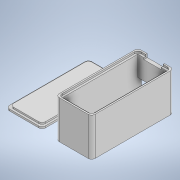
# Autodesk Inventor part: case
Saved by Autodesk Inventor 2021 (Build 250183000, 183)
## iProperties
Created: 2021-06-14
Part Number: case
Material: 일반
Document SubType Name: Modeling
Designer: dltjd
Density: 1 g/cm^3
Appearance: 기본값
Author: dltjd
Autodesk Inventor part; units mm, degrees
ref_plane "YZ Plane" through (0, 0, 0) normal (1, 0, 0) x (0, 1, 0)
ref_plane "XZ Plane" through (0, 0, 0) normal (0, 1, 0) x (-1, 0, 0)
ref_plane "XY Plane" through (0, 0, 0) normal (0, 0, 1) x (1, 0, 0)
sketch "스케치1" plane through (0, 0, 0) normal (0, 1, 0) x (-1, 0, 0)
  line L0 (14, 34) -> (-14, 34)
  line L1 (-14, 34) -> (-14, -34)
  line L2 (-14, -34) -> (14, -34)
  line L3 (14, -34) -> (14, 34)
  line L4 (14, 34) -> (-14, -34) construction
  line L5 (-14, 34) -> (14, -34) construction
  point P0 (0, 0)
  dimension "d0" = 28
  dimension "d1" = 68
  constraints: 12 end point, 2 midpoint, 2 parallel, 1 horizontal, 1 perpendicular
  measures "d0" distance of L2.end L1.end
  measures "d1" distance of L1.end L0.end
extrude "돌출1" add sketch "스케치1" along normal blind 1.5
sketch "스케치2" plane through (0, 1.5, 0) normal (0, 1, 0) x (1, 0, 0)
  line L0 (-14, 34) -> (-14, -34) projected
  line L1 (14, -34) -> (14, 34) projected
  line L2 (-14, -34) -> (14, -34)
  line L3 (14, -34) -> (14, -32.5)
  line L4 (14, -32.5) -> (-14, -32.5)
  line L5 (-14, -32.5) -> (-14, -34)
  line L6 (14, 34) -> (-14, 34) projected
  line L7 (-14, -34) -> (-12.5, -34)
  line L8 (-12.5, -34) -> (-12.5, 34)
  line L9 (-12.5, 34) -> (-14, 34)
  line L10 (-14, 34) -> (-14, -34)
  line L11 (14, -34) -> (12.5, -34)
  line L12 (12.5, -34) -> (12.5, 34)
  line L13 (12.5, 34) -> (14, 34)
  line L14 (14, 34) -> (14, -34)
  point P0 (0, 0)
  point P1 (12.5, -32.5)
  point P2 (-12.5, -32.5)
  dimension "d4" = 1.5
  dimension "d5" = 1.5
  dimension "d6" = 1.5
  constraints: 24 end point, 6 parallel, 3 horizontal, 3 perpendicular, 3 point on line
  measures "d4" distance of L3.end L2.end
  measures "d5" distance of L9.end L8.end
  measures "d6" distance of L12.end L13.end
extrude "돌출2" add sketch "스케치2" along normal blind 30 contours L6 L8 L4 L0 | L4 L8 L2 L0 | L4 L12 L2 L8 | L6 L1 L4 L12 | L4 L1 L2 L12
sketch "스케치3" plane through (0, 1.5, 0) normal (0, 1, 0) x (1, 0, 0)
  line L0 (-14, 34) -> (-14, -34) projected
  line L1 (14, -34) -> (14, 34) projected
  line L2 (-14, 34) -> (14, 34)
  line L3 (14, 34) -> (14, 32.5)
  line L4 (14, 32.5) -> (-14, 32.5)
  line L5 (-14, 32.5) -> (-14, 34)
  point P0 (0, 0)
  dimension "d9" = 1.5
  constraints: 8 end point, 2 parallel, 1 horizontal, 1 perpendicular, 1 point on line
  measures "d9" distance of L2.end L3.end
extrude "돌출3" add sketch "스케치3" along normal blind 30
sketch "스케치5" plane through (0, 1.5, 0) normal (0, 1, 0) x (1, 0, 0)
  line L0 (-27.2681, 35.5) -> (-58.2681, 35.5)
  line L1 (-58.2681, 35.5) -> (-58.2681, -35.5)
  line L2 (-58.2681, -35.5) -> (-27.2681, -35.5)
  line L3 (-27.2681, -35.5) -> (-27.2681, 35.5)
  line L4 (-27.2681, 35.5) -> (-58.2681, -35.5) construction
  line L5 (-58.2681, 35.5) -> (-27.2681, -35.5) construction
  point P0 (0, 0)
  point P1 (-42.7681, 0)
  dimension "d36" = 31
  dimension "d37" = 71
  constraints: 12 end point, 2 midpoint, 2 parallel, 1 horizontal, 1 perpendicular
  measures "d36" distance of L2.end L1.end
  measures "d37" distance of L1.end L0.end
ref_plane "작업 평면1" through (0, 3, 0) normal (0, 1, 0) x (1, 0, 0)
sketch "스케치7" plane through (14, 0, -34) normal (0, 0, -1) x (-1, 0, 0)
  line L0 (0, 31.5) -> (28, 31.5) projected
  line L1 (0, 31.5) -> (28, 31.5)
  line L2 (28, 31.5) -> (28, 0)
  line L3 (28, 0) -> (0, 0)
  line L4 (0, 0) -> (0, 31.5)
  point P0 (14, 0)
  constraints: 8 end point, 2 parallel, 1 horizontal, 1 perpendicular
extrude "돌출7" add sketch "스케치7" along normal blind 1.5
sketch "스케치8" plane through (0, 1.5, 0) normal (0, 1, 0) x (1, 0, 0)
  line L0 (12.5, 32.5) -> (12.5, -32.5) projected
  line L1 (14, 35.5) -> (-14, 35.5) projected
  line L2 (12.5, 32.5) -> (-12.5, 32.5)
  line L3 (-12.5, 32.5) -> (-12.5, 35.5)
  line L4 (-12.5, 35.5) -> (12.5, 35.5)
  line L5 (12.5, 35.5) -> (12.5, 32.5)
  point P0 (0, 0)
  dimension "d26" = 25
  constraints: 8 end point, 2 parallel, 1 horizontal, 1 perpendicular, 1 point on line
  measures "d26" distance of L3.end L4.end
sketch "스케치9" plane through (14, 0, 34) normal (1, 0, 0) x (0, 0, -1)
  line L0 (0, 31.5) -> (69.5, 31.5) projected
  line L1 (69.5, 31.5) -> (0, 31.5)
  line L2 (0, 31.5) -> (0, 0)
  line L3 (0, 0) -> (69.5, 0)
  line L4 (69.5, 0) -> (69.5, 31.5)
  point P0 (34, 0)
  constraints: 8 end point, 2 parallel, 1 horizontal, 1 perpendicular
extrude "돌출9" add sketch "스케치9" along normal blind 1.5
sketch "스케치10" plane through (-14, 0, 34) normal (0, 0, 1) x (1, 0, 0)
  line L0 (0, 0) -> (0, 31.5) projected
  line L1 (29.5, 31.5) -> (29.5, 0) projected
  line L2 (0, 31.5) -> (29.5, 31.5)
  line L3 (29.5, 31.5) -> (29.5, 0)
  line L4 (29.5, 0) -> (0, 0)
  line L5 (0, 0) -> (0, 31.5)
  point P0 (14, 0)
  constraints: 8 end point, 2 parallel, 1 horizontal, 1 perpendicular
extrude "돌출10" add sketch "스케치10" along normal blind 1.5
sketch "스케치11" plane through (-14, 0, -35.5) normal (-1, 0, 0) x (0, 0, 1)
  line L0 (0, 31.5) -> (71, 31.5) projected
  line L1 (0, 0) -> (71, 0)
  line L2 (71, 0) -> (71, 31.5)
  line L3 (71, 31.5) -> (0, 31.5)
  line L4 (0, 31.5) -> (0, 0)
  point P0 (35.5, 0)
  constraints: 8 end point, 2 parallel, 1 horizontal, 1 perpendicular
extrude "돌출11" add sketch "스케치11" along normal blind 1.5
fillet "모깎기1" radius 3 4 edges at (15.5, 15.75, -35.5) (-15.5, 15.75, -35.5) (-15.5, 15.75, 35.5) (15.5, 15.75, 35.5)
extrude "돌출12" add sketch "스케치5" along normal blind 1.5
fillet "모깎기2" radius 3 4 edges at (-58.2681, 2.25, 35.5) (-27.2681, 2.25, 35.5) (-27.2681, 2.25, -35.5) (-58.2681, 2.25, -35.5)
sketch "스케치12" plane through (0, 31.5, 0) normal (0, 1, 0) x (1, 0, 0)
  line L0 (-14, -31.6724) -> (-14, -27.7757)
  line L1 (14, 29.0808) -> (14, 30.2026)
  line L2 (-12.5, 32.5) -> (12.5, 32.5) projected
  line L3 (7.6672, 32.5) -> (14, 32.5)
  line L4 (-11, -34) -> (11, -34)
  line L5 (14, -31) -> (14, 31)
  line L6 (11, 34) -> (-11, 34)
  line L7 (-14, 31) -> (-14, -31)
  line L8 (-12.5, -35.5) -> (12.5, -35.5)
  line L9 (15.5, -32.5) -> (15.5, 32.5)
  line L10 (12.5, 35.5) -> (-12.5, 35.5)
  line L11 (-15.5, 32.5) -> (-15.5, -32.5)
  arc A0 (-15.5, -32.5) -> (-12.5, -35.5) centre (-12.5, -32.5) ccw
  arc A1 (12.5, -35.5) -> (15.5, -32.5) centre (12.5, -32.5) ccw
  arc A2 (15.5, 32.5) -> (12.5, 35.5) centre (12.5, 32.5) ccw
  arc A3 (-12.5, 35.5) -> (-15.5, 32.5) centre (-12.5, 32.5) ccw
  arc A4 (14, 31) -> (11, 34) centre (11, 31) ccw
  arc A5 (-11, 34) -> (-14, 31) centre (-11, 31) ccw
  arc A6 (-14, -31) -> (-11, -34) centre (-11, -31) ccw
  arc A7 (11, -34) -> (14, -31) centre (11, -31) ccw
  point P0 (0, 0)
  dimension "d45" = 3
  constraints: 22 end point, 16 point on circle, 16 tangent, 8 centre point, 7 equal radius, 4 parallel, 3 horizontal, 2 perpendicular, 1 point on line
  measures "d45" radius of A0
extrude "돌출13" add sketch "스케치12" along normal blind 1.5
sketch "스케치13" plane through (0, 3, 0) normal (0, 1, 0) x (1, 0, 0)
  line L0 (-56.5181, -11.0824) -> (-56.5181, -10.5346)
  line L1 (-43.8335, -33.75) -> (-45.2942, -33.75)
  line L2 (-29.0181, -15.4369) -> (-29.0181, -13.7413)
  line L3 (-44.3798, 33.75) -> (-42.3798, 33.75)
  line L4 (-53.5181, -33.75) -> (-32.0181, -33.75)
  line L5 (-29.0181, -30.75) -> (-29.0181, 30.75)
  line L6 (-32.0181, 33.75) -> (-53.5181, 33.75)
  line L7 (-56.5181, 30.75) -> (-56.5181, -30.75)
  arc A0 (-56.5181, -30.75) -> (-53.5181, -33.75) centre (-53.5181, -30.75) ccw
  arc A1 (-32.0181, -33.75) -> (-29.0181, -30.75) centre (-32.0181, -30.75) ccw
  arc A2 (-29.0181, 30.75) -> (-32.0181, 33.75) centre (-32.0181, 30.75) ccw
  arc A3 (-53.5181, 33.75) -> (-56.5181, 30.75) centre (-53.5181, 30.75) ccw
  point P0 (0, 0)
  point P1 (-56.7681, -34)
  point P2 (-28.7681, 34)
  point P3 (-29.0181, 33.75)
  dimension "d76" = 3
  constraints: 16 end point, 8 point on circle, 8 tangent, 4 centre point, 4 point on line, 3 equal radius, 2 parallel, 1 horizontal, 1 perpendicular
  measures "d76" radius of A0
sketch "스케치14" plane through (0, 1.5, 0) normal (0, -1, 0) x (1, 0, 0)
  line L0 (-44.3921, -14.3977) -> (-44.3921, 14.3977) construction
  line L1 (-44.3921, 14.3977) -> (-41.144, 14.3977) construction
  line L2 (-41.144, 14.3977) -> (-41.144, -14.3977) construction
  line L3 (-41.144, -14.3977) -> (-44.3921, -14.3977) construction
  line L4 (-30.2681, -35.5) -> (-55.2681, -35.5) projected
  line L5 (-58.2681, -32.5) -> (-58.2681, 32.5) projected
  line L6 (-41.7389, -11.7877) -> (-41.7389, -12.5637)
  line L7 (-41.7389, -12.5637) -> (-42.6713, -13.2698)
  line L8 (-42.6713, -13.2698) -> (-42.6713, -13.5003)
  line L9 (-42.6713, -13.5003) -> (-41.7389, -13.5003)
  line L10 (-41.7389, -13.5003) -> (-41.7389, -14.1343)
  line L11 (-41.7389, -14.1343) -> (-44.2789, -14.1343)
  line L12 (-44.2789, -14.1343) -> (-44.2789, -13.1133)
  spline S0 degree 2 poles (-44.2789, -13.1133) (-44.2789, -12.9013) (-44.2254, -12.5884) (-44.1431, -12.4546) knots 0 0 0 1 2 2 2
  spline S1 degree 2 poles (-44.1431, -12.4546) (-44.0566, -12.3188) (-43.787, -12.1582) (-43.5811, -12.1582) knots 0 0 0 1 2 2 2
  spline S2 degree 2 poles (-43.5811, -12.1582) (-43.2909, -12.1582) (-42.9266, -12.4217) (-42.8195, -12.642) knots 0 0 0 1 2 2 2
  line L13 (-42.8195, -12.642) -> (-41.7389, -11.7877)
  spline S3 degree 2 poles (-43.5009, -12.8128) (-43.5976, -12.8128) (-43.7355, -12.8869) (-43.7726, -12.9713) knots 0 0 0 1 2 2 2
  spline S4 degree 2 poles (-43.7726, -12.9713) (-43.7973, -13.031) (-43.8117, -13.1771) (-43.8117, -13.2862) knots 0 0 0 1 2 2 2
  line L14 (-43.8117, -13.2862) -> (-43.8117, -13.5003)
  line L15 (-43.8117, -13.5003) -> (-43.1283, -13.5003)
  line L16 (-43.1283, -13.5003) -> (-43.1283, -13.3171)
  spline S5 degree 2 poles (-43.1283, -13.3171) (-43.1283, -13.1854) (-43.1612, -12.998) (-43.2127, -12.9342) knots 0 0 0 1 2 2 2
  spline S6 degree 2 poles (-43.2127, -12.9342) (-43.2621, -12.8725) (-43.3938, -12.8128) (-43.5009, -12.8128) knots 0 0 0 1 2 2 2
  spline S7 degree 2 poles (-41.6874, -10.6515) (-41.6874, -11.1949) (-42.2062, -11.7733) (-42.6857, -11.7733) knots 0 0 0 1 2 2 2
  spline S8 degree 2 poles (-42.6857, -11.7733) (-43.1551, -11.7733) (-43.7149, -11.234) (-43.7149, -10.7483) knots 0 0 0 1 2 2 2
  spline S9 degree 2 poles (-43.7149, -10.7483) (-43.7149, -10.3098) (-43.2394, -9.8652) (-42.799, -9.8652) knots 0 0 0 1 2 2 2
  line L17 (-42.799, -9.8652) -> (-42.5828, -9.8652)
  line L18 (-42.5828, -9.8652) -> (-42.5828, -11.1764)
  spline S10 degree 2 poles (-42.5828, -11.1764) (-42.449, -11.1682) (-42.272, -11.0714) (-42.2185, -10.9932) knots 0 0 0 1 2 2 2
  spline S11 degree 2 poles (-42.2185, -10.9932) (-42.165, -10.9171) (-42.1197, -10.7112) (-42.1197, -10.5898) knots 0 0 0 1 2 2 2
  spline S12 degree 2 poles (-42.1197, -10.5898) (-42.1197, -10.4869) (-42.165, -10.2851) (-42.2041, -10.2008) knots 0 0 0 1 2 2 2
  spline S13 degree 2 poles (-42.2041, -10.2008) (-42.235, -10.1267) (-42.3111, -10.0032) (-42.3399, -9.964) knots 0 0 0 1 2 2 2
  line L19 (-42.3399, -9.964) -> (-42.3399, -9.9002)
  line L20 (-42.3399, -9.9002) -> (-41.8459, -9.9002)
  spline S14 degree 2 poles (-41.8459, -9.9002) (-41.8171, -9.9743) (-41.7677, -10.0937) (-41.743, -10.2008) knots 0 0 0 1 2 2 2
  spline S15 degree 2 poles (-41.743, -10.2008) (-41.7163, -10.2975) (-41.6874, -10.5033) (-41.6874, -10.6515) knots 0 0 0 1 2 2 2
  spline S16 degree 2 poles (-42.943, -10.4539) (-43.1324, -10.458) (-43.3321, -10.6248) (-43.3321, -10.7956) knots 0 0 0 1 2 2 2
  spline S17 degree 2 poles (-43.3321, -10.7956) (-43.3321, -10.9706) (-43.1221, -11.1682) (-42.943, -11.1785) knots 0 0 0 1 2 2 2
  line L21 (-42.943, -11.1785) -> (-42.943, -10.4539)
  line L22 (-41.7389, -7.2717) -> (-42.696, -7.2717)
  spline S18 degree 2 poles (-42.696, -7.2717) (-42.8381, -7.2717) (-43.0315, -7.282) (-43.0933, -7.3067) knots 0 0 0 1 2 2 2
  spline S19 degree 2 poles (-43.0933, -7.3067) (-43.1551, -7.3335) (-43.2106, -7.4405) (-43.2106, -7.5373) knots 0 0 0 1 2 2 2
  spline S20 degree 2 poles (-43.2106, -7.5373) (-43.2106, -7.6052) (-43.1509, -7.7369) (-43.0954, -7.8151) knots 0 0 0 1 2 2 2
  line L23 (-43.0954, -7.8151) -> (-41.7389, -7.8151)
  line L24 (-41.7389, -7.8151) -> (-41.7389, -8.4162)
  line L25 (-41.7389, -8.4162) -> (-42.696, -8.4162)
  spline S21 degree 2 poles (-42.696, -8.4162) (-42.836, -8.4162) (-43.0315, -8.4285) (-43.0933, -8.4532) knots 0 0 0 1 2 2 2
  spline S22 degree 2 poles (-43.0933, -8.4532) (-43.1551, -8.48) (-43.2106, -8.587) (-43.2106, -8.6838) knots 0 0 0 1 2 2 2
  spline S23 degree 2 poles (-43.2106, -8.6838) (-43.2106, -8.7558) (-43.1427, -8.8978) (-43.0954, -8.9637) knots 0 0 0 1 2 2 2
  line L26 (-43.0954, -8.9637) -> (-41.7389, -8.9637)
  line L27 (-41.7389, -8.9637) -> (-41.7389, -9.5606)
  line L28 (-41.7389, -9.5606) -> (-43.6552, -9.5606)
  line L29 (-43.6552, -9.5606) -> (-43.6552, -8.9637)
  line L30 (-43.6552, -8.9637) -> (-43.4432, -8.9637)
  spline S24 degree 2 poles (-43.4432, -8.9637) (-43.5667, -8.8175) (-43.7067, -8.5561) (-43.7067, -8.3935) knots 0 0 0 1 2 2 2
  spline S25 degree 2 poles (-43.7067, -8.3935) (-43.7067, -8.2186) (-43.54, -7.951) (-43.3732, -7.881) knots 0 0 0 1 2 2 2
  spline S26 degree 2 poles (-43.3732, -7.881) (-43.5338, -7.7102) (-43.7067, -7.4055) (-43.7067, -7.2491) knots 0 0 0 1 2 2 2
  spline S27 degree 2 poles (-43.7067, -7.2491) (-43.7067, -7.1153) (-43.6223, -6.9033) (-43.5358, -6.8312) knots 0 0 0 1 2 2 2
  spline S28 degree 2 poles (-43.5358, -6.8312) (-43.4432, -6.751) (-43.19, -6.6707) (-42.9863, -6.6707) knots 0 0 0 1 2 2 2
  line L31 (-42.9863, -6.6707) -> (-41.7389, -6.6707)
  line L32 (-41.7389, -6.6707) -> (-41.7389, -7.2717)
  spline S29 degree 2 poles (-42.696, -4.39) (-42.2226, -4.39) (-41.6792, -4.9067) (-41.6792, -5.378) knots 0 0 0 1 2 2 2
  spline S30 degree 2 poles (-41.6792, -5.378) (-41.6792, -5.8474) (-42.2226, -6.3681) (-42.696, -6.3681) knots 0 0 0 1 2 2 2
  spline S31 degree 2 poles (-42.696, -6.3681) (-43.1736, -6.3681) (-43.7149, -5.8474) (-43.7149, -5.378) knots 0 0 0 1 2 2 2
  spline S32 degree 2 poles (-43.7149, -5.378) (-43.7149, -4.9087) (-43.1715, -4.39) (-42.696, -4.39) knots 0 0 0 1 2 2 2
  spline S33 degree 2 poles (-42.6919, -5.0014) (-42.8628, -5.0014) (-43.0912, -5.0569) (-43.1592, -5.1063) knots 0 0 0 1 2 2 2
  spline S34 degree 2 poles (-43.1592, -5.1063) (-43.2312, -5.1599) (-43.2868, -5.2937) (-43.2868, -5.378) knots 0 0 0 1 2 2 2
  spline S35 degree 2 poles (-43.2868, -5.378) (-43.2868, -5.4604) (-43.2374, -5.5901) (-43.1674, -5.6436) knots 0 0 0 1 2 2 2
  spline S36 degree 2 poles (-43.1674, -5.6436) (-43.1015, -5.695) (-42.8689, -5.7568) (-42.6919, -5.7568) knots 0 0 0 1 2 2 2
  spline S37 degree 2 poles (-42.6919, -5.7568) (-42.517, -5.7568) (-42.3008, -5.6992) (-42.235, -5.6518) knots 0 0 0 1 2 2 2
  spline S38 degree 2 poles (-42.235, -5.6518) (-42.1691, -5.6045) (-42.1074, -5.4604) (-42.1074, -5.3739) knots 0 0 0 1 2 2 2
  spline S39 degree 2 poles (-42.1074, -5.3739) (-42.1074, -5.3019) (-42.1691, -5.1537) (-42.2309, -5.1084) knots 0 0 0 1 2 2 2
  spline S40 degree 2 poles (-42.2309, -5.1084) (-42.3029, -5.0569) (-42.5108, -5.0014) (-42.6919, -5.0014) knots 0 0 0 1 2 2 2
  spline S41 degree 2 poles (-41.7019, -3.3403) (-41.7019, -3.7046) (-42.0024, -4.0381) (-42.3441, -4.0381) knots 0 0 0 1 2 2 2
  line L33 (-42.3441, -4.0381) -> (-43.2394, -4.0381)
  line L34 (-43.2394, -4.0381) -> (-43.2394, -4.2665)
  line L35 (-43.2394, -4.2665) -> (-43.6552, -4.2665)
  line L36 (-43.6552, -4.2665) -> (-43.6552, -4.0381)
  line L37 (-43.6552, -4.0381) -> (-44.2027, -4.0381)
  line L38 (-44.2027, -4.0381) -> (-44.2027, -3.4411)
  line L39 (-44.2027, -3.4411) -> (-43.6552, -3.4411)
  line L40 (-43.6552, -3.4411) -> (-43.6552, -2.8648)
  line L41 (-43.6552, -2.8648) -> (-43.2394, -2.8648)
  line L42 (-43.2394, -2.8648) -> (-43.2394, -3.4411)
  line L43 (-43.2394, -3.4411) -> (-42.5581, -3.4411)
  spline S42 degree 2 poles (-42.5581, -3.4411) (-42.4573, -3.4411) (-42.307, -3.437) (-42.2473, -3.4123) knots 0 0 0 1 2 2 2
  spline S43 degree 2 poles (-42.2473, -3.4123) (-42.1876, -3.3876) (-42.1176, -3.2662) (-42.1176, -3.1509) knots 0 0 0 1 2 2 2
  spline S44 degree 2 poles (-42.1176, -3.1509) (-42.1176, -3.1015) (-42.1588, -2.9471) (-42.1753, -2.9163) knots 0 0 0 1 2 2 2
  line L44 (-42.1753, -2.9163) -> (-42.1753, -2.8648)
  line L45 (-42.1753, -2.8648) -> (-41.7554, -2.8648)
  spline S45 degree 2 poles (-41.7554, -2.8648) (-41.7307, -2.9615) (-41.7019, -3.1797) (-41.7019, -3.3403) knots 0 0 0 1 2 2 2
  spline S46 degree 2 poles (-41.6874, -1.6401) (-41.6874, -2.1835) (-42.2062, -2.7619) (-42.6857, -2.7619) knots 0 0 0 1 2 2 2
  spline S47 degree 2 poles (-42.6857, -2.7619) (-43.1551, -2.7619) (-43.7149, -2.2226) (-43.7149, -1.7368) knots 0 0 0 1 2 2 2
  spline S48 degree 2 poles (-43.7149, -1.7368) (-43.7149, -1.2984) (-43.2394, -0.8538) (-42.799, -0.8538) knots 0 0 0 1 2 2 2
  line L46 (-42.799, -0.8538) -> (-42.5828, -0.8538)
  line L47 (-42.5828, -0.8538) -> (-42.5828, -2.165)
  spline S49 degree 2 poles (-42.5828, -2.165) (-42.449, -2.1567) (-42.272, -2.06) (-42.2185, -1.9818) knots 0 0 0 1 2 2 2
  spline S50 degree 2 poles (-42.2185, -1.9818) (-42.165, -1.9056) (-42.1197, -1.6998) (-42.1197, -1.5783) knots 0 0 0 1 2 2 2
  spline S51 degree 2 poles (-42.1197, -1.5783) (-42.1197, -1.4754) (-42.165, -1.2737) (-42.2041, -1.1893) knots 0 0 0 1 2 2 2
  spline S52 degree 2 poles (-42.2041, -1.1893) (-42.235, -1.1152) (-42.3111, -0.9917) (-42.3399, -0.9526) knots 0 0 0 1 2 2 2
  line L48 (-42.3399, -0.9526) -> (-42.3399, -0.8888)
  line L49 (-42.3399, -0.8888) -> (-41.8459, -0.8888)
  spline S53 degree 2 poles (-41.8459, -0.8888) (-41.8171, -0.9629) (-41.7677, -1.0823) (-41.743, -1.1893) knots 0 0 0 1 2 2 2
  spline S54 degree 2 poles (-41.743, -1.1893) (-41.7163, -1.2861) (-41.6874, -1.4919) (-41.6874, -1.6401) knots 0 0 0 1 2 2 2
  spline S55 degree 2 poles (-42.943, -1.4425) (-43.1324, -1.4466) (-43.3321, -1.6133) (-43.3321, -1.7842) knots 0 0 0 1 2 2 2
  spline S56 degree 2 poles (-43.3321, -1.7842) (-43.3321, -1.9591) (-43.1221, -2.1567) (-42.943, -2.167) knots 0 0 0 1 2 2 2
  line L50 (-42.943, -2.167) -> (-42.943, -1.4425)
  spline S57 degree 2 poles (-41.6895, 1.6059) (-41.6895, 1.0337) (-42.3811, 0.3627) (-43.0068, 0.3627) knots 0 0 0 1 2 2 2
  spline S58 degree 2 poles (-43.0068, 0.3627) (-43.6099, 0.3627) (-44.3283, 1.0358) (-44.3283, 1.608) knots 0 0 0 1 2 2 2
  spline S59 degree 2 poles (-44.3283, 1.608) (-44.3283, 1.7582) (-44.2933, 2.0011) (-44.2645, 2.1123) knots 0 0 0 1 2 2 2
  spline S60 degree 2 poles (-44.2645, 2.1123) (-44.2377, 2.1987) (-44.1492, 2.4025) (-44.1163, 2.4663) knots 0 0 0 1 2 2 2
  line L51 (-44.1163, 2.4663) -> (-43.5111, 2.4663)
  line L52 (-43.5111, 2.4663) -> (-43.5111, 2.4025)
  spline S61 degree 2 poles (-43.5111, 2.4025) (-43.5523, 2.3552) (-43.6676, 2.2152) (-43.7211, 2.1267) knots 0 0 0 1 2 2 2
  spline S62 degree 2 poles (-43.7211, 2.1267) (-43.7767, 2.0382) (-43.8528, 1.8262) (-43.8528, 1.7088) knots 0 0 0 1 2 2 2
  spline S63 degree 2 poles (-43.8528, 1.7088) (-43.8528, 1.5709) (-43.7664, 1.3425) (-43.6573, 1.2375) knots 0 0 0 1 2 2 2
  spline S64 degree 2 poles (-43.6573, 1.2375) (-43.5605, 1.1428) (-43.2292, 1.0214) (-43.0048, 1.0214) knots 0 0 0 1 2 2 2
  spline S65 degree 2 poles (-43.0048, 1.0214) (-42.7681, 1.0214) (-42.4449, 1.1469) (-42.3461, 1.2498) knots 0 0 0 1 2 2 2
  spline S66 degree 2 poles (-42.3461, 1.2498) (-42.2494, 1.3486) (-42.165, 1.5915) (-42.165, 1.713) knots 0 0 0 1 2 2 2
  spline S67 degree 2 poles (-42.165, 1.713) (-42.165, 1.8385) (-42.2494, 2.067) (-42.3008, 2.1452) knots 0 0 0 1 2 2 2
  spline S68 degree 2 poles (-42.3008, 2.1452) (-42.3523, 2.2317) (-42.4614, 2.3613) (-42.5046, 2.4087) knots 0 0 0 1 2 2 2
  line L53 (-42.5046, 2.4087) -> (-42.5046, 2.4663)
  line L54 (-42.5046, 2.4663) -> (-41.9077, 2.4663)
  spline S69 degree 2 poles (-41.9077, 2.4663) (-41.8748, 2.3963) (-41.7924, 2.2131) (-41.7636, 2.1143) knots 0 0 0 1 2 2 2
  spline S70 degree 2 poles (-41.7636, 2.1143) (-41.7266, 1.9949) (-41.6895, 1.7871) (-41.6895, 1.6059) knots 0 0 0 1 2 2 2
  spline S71 degree 2 poles (-42.696, 4.6461) (-42.2226, 4.6461) (-41.6792, 4.1295) (-41.6792, 3.6581) knots 0 0 0 1 2 2 2
  spline S72 degree 2 poles (-41.6792, 3.6581) (-41.6792, 3.1888) (-42.2226, 2.668) (-42.696, 2.668) knots 0 0 0 1 2 2 2
  spline S73 degree 2 poles (-42.696, 2.668) (-43.1736, 2.668) (-43.7149, 3.1888) (-43.7149, 3.6581) knots 0 0 0 1 2 2 2
  spline S74 degree 2 poles (-43.7149, 3.6581) (-43.7149, 4.1274) (-43.1715, 4.6461) (-42.696, 4.6461) knots 0 0 0 1 2 2 2
  spline S75 degree 2 poles (-42.6919, 4.0348) (-42.8628, 4.0348) (-43.0912, 3.9792) (-43.1592, 3.9298) knots 0 0 0 1 2 2 2
  spline S76 degree 2 poles (-43.1592, 3.9298) (-43.2312, 3.8763) (-43.2868, 3.7425) (-43.2868, 3.6581) knots 0 0 0 1 2 2 2
  spline S77 degree 2 poles (-43.2868, 3.6581) (-43.2868, 3.5758) (-43.2374, 3.4461) (-43.1674, 3.3926) knots 0 0 0 1 2 2 2
  spline S78 degree 2 poles (-43.1674, 3.3926) (-43.1015, 3.3411) (-42.8689, 3.2794) (-42.6919, 3.2794) knots 0 0 0 1 2 2 2
  spline S79 degree 2 poles (-42.6919, 3.2794) (-42.517, 3.2794) (-42.3008, 3.337) (-42.235, 3.3843) knots 0 0 0 1 2 2 2
  spline S80 degree 2 poles (-42.235, 3.3843) (-42.1691, 3.4317) (-42.1074, 3.5758) (-42.1074, 3.6622) knots 0 0 0 1 2 2 2
  spline S81 degree 2 poles (-42.1074, 3.6622) (-42.1074, 3.7343) (-42.1691, 3.8825) (-42.2309, 3.9277) knots 0 0 0 1 2 2 2
  spline S82 degree 2 poles (-42.2309, 3.9277) (-42.3029, 3.9792) (-42.5108, 4.0348) (-42.6919, 4.0348) knots 0 0 0 1 2 2 2
  line L55 (-41.7389, 6.7559) -> (-41.7389, 6.1549)
  line L56 (-41.7389, 6.1549) -> (-42.6878, 6.1549)
  spline S83 degree 2 poles (-42.6878, 6.1549) (-42.8051, 6.1549) (-43.0357, 6.1363) (-43.0892, 6.1116) knots 0 0 0 1 2 2 2
  spline S84 degree 2 poles (-43.0892, 6.1116) (-43.1551, 6.0808) (-43.2106, 5.9655) (-43.2106, 5.8667) knots 0 0 0 1 2 2 2
  spline S85 degree 2 poles (-43.2106, 5.8667) (-43.2106, 5.7947) (-43.1551, 5.6444) (-43.0954, 5.56) knots 0 0 0 1 2 2 2
  line L57 (-43.0954, 5.56) -> (-41.7389, 5.56)
  line L58 (-41.7389, 5.56) -> (-41.7389, 4.9631)
  line L59 (-41.7389, 4.9631) -> (-43.6552, 4.9631)
  line L60 (-43.6552, 4.9631) -> (-43.6552, 5.56)
  line L61 (-43.6552, 5.56) -> (-43.4432, 5.56)
  spline S86 degree 2 poles (-43.4432, 5.56) (-43.5667, 5.7061) (-43.7067, 5.984) (-43.7067, 6.1528) knots 0 0 0 1 2 2 2
  spline S87 degree 2 poles (-43.7067, 6.1528) (-43.7067, 6.4451) (-43.3362, 6.7559) (-42.9863, 6.7559) knots 0 0 0 1 2 2 2
  line L62 (-42.9863, 6.7559) -> (-41.7389, 6.7559)
  spline S88 degree 2 poles (-41.7019, 7.9312) (-41.7019, 7.5669) (-42.0024, 7.2334) (-42.3441, 7.2334) knots 0 0 0 1 2 2 2
  line L63 (-42.3441, 7.2334) -> (-43.2394, 7.2334)
  line L64 (-43.2394, 7.2334) -> (-43.2394, 7.005)
  line L65 (-43.2394, 7.005) -> (-43.6552, 7.005)
  line L66 (-43.6552, 7.005) -> (-43.6552, 7.2334)
  line L67 (-43.6552, 7.2334) -> (-44.2027, 7.2334)
  line L68 (-44.2027, 7.2334) -> (-44.2027, 7.8304)
  line L69 (-44.2027, 7.8304) -> (-43.6552, 7.8304)
  line L70 (-43.6552, 7.8304) -> (-43.6552, 8.4067)
  line L71 (-43.6552, 8.4067) -> (-43.2394, 8.4067)
  line L72 (-43.2394, 8.4067) -> (-43.2394, 7.8304)
  line L73 (-43.2394, 7.8304) -> (-42.5581, 7.8304)
  spline S89 degree 2 poles (-42.5581, 7.8304) (-42.4573, 7.8304) (-42.307, 7.8345) (-42.2473, 7.8592) knots 0 0 0 1 2 2 2
  spline S90 degree 2 poles (-42.2473, 7.8592) (-42.1876, 7.8839) (-42.1176, 8.0053) (-42.1176, 8.1206) knots 0 0 0 1 2 2 2
  spline S91 degree 2 poles (-42.1176, 8.1206) (-42.1176, 8.17) (-42.1588, 8.3244) (-42.1753, 8.3552) knots 0 0 0 1 2 2 2
  line L74 (-42.1753, 8.3552) -> (-42.1753, 8.4067)
  line L75 (-42.1753, 8.4067) -> (-41.7554, 8.4067)
  spline S92 degree 2 poles (-41.7554, 8.4067) (-41.7307, 8.31) (-41.7019, 8.0918) (-41.7019, 7.9312) knots 0 0 0 1 2 2 2
  line L76 (-43.0892, 9.9361) -> (-43.0892, 9.8867)
  spline S93 degree 2 poles (-43.0892, 9.8867) (-43.1015, 9.8517) (-43.1139, 9.722) (-43.1139, 9.6438) knots 0 0 0 1 2 2 2
  spline S94 degree 2 poles (-43.1139, 9.6438) (-43.1139, 9.5511) (-43.0583, 9.3432) (-43.0213, 9.2465) knots 0 0 0 1 2 2 2
  line L77 (-43.0213, 9.2465) -> (-41.7389, 9.2465)
  line L78 (-41.7389, 9.2465) -> (-41.7389, 8.6496)
  line L79 (-41.7389, 8.6496) -> (-43.6552, 8.6496)
  line L80 (-43.6552, 8.6496) -> (-43.6552, 9.2465)
  line L81 (-43.6552, 9.2465) -> (-43.3794, 9.2465)
  spline S95 degree 2 poles (-43.3794, 9.2465) (-43.4165, 9.2877) (-43.5317, 9.4318) (-43.5667, 9.4914) knots 0 0 0 1 2 2 2
  spline S96 degree 2 poles (-43.5667, 9.4914) (-43.6058, 9.5573) (-43.6614, 9.7302) (-43.6614, 9.8064) knots 0 0 0 1 2 2 2
  spline S97 degree 2 poles (-43.6614, 9.8064) (-43.6614, 9.8352) (-43.6573, 9.9072) (-43.6552, 9.9361) knots 0 0 0 1 2 2 2
  line L82 (-43.6552, 9.9361) -> (-43.0892, 9.9361)
  spline S98 degree 2 poles (-42.696, 12.0026) (-42.2226, 12.0026) (-41.6792, 11.486) (-41.6792, 11.0146) knots 0 0 0 1 2 2 2
  spline S99 degree 2 poles (-41.6792, 11.0146) (-41.6792, 10.5453) (-42.2226, 10.0246) (-42.696, 10.0246) knots 0 0 0 1 2 2 2
  spline S100 degree 2 poles (-42.696, 10.0246) (-43.1736, 10.0246) (-43.7149, 10.5453) (-43.7149, 11.0146) knots 0 0 0 1 2 2 2
  spline S101 degree 2 poles (-43.7149, 11.0146) (-43.7149, 11.4839) (-43.1715, 12.0026) (-42.696, 12.0026) knots 0 0 0 1 2 2 2
  spline S102 degree 2 poles (-42.6919, 11.3913) (-42.8628, 11.3913) (-43.0912, 11.3357) (-43.1592, 11.2863) knots 0 0 0 1 2 2 2
  spline S103 degree 2 poles (-43.1592, 11.2863) (-43.2312, 11.2328) (-43.2868, 11.099) (-43.2868, 11.0146) knots 0 0 0 1 2 2 2
  spline S104 degree 2 poles (-43.2868, 11.0146) (-43.2868, 10.9323) (-43.2374, 10.8026) (-43.1674, 10.7491) knots 0 0 0 1 2 2 2
  spline S105 degree 2 poles (-43.1674, 10.7491) (-43.1015, 10.6976) (-42.8689, 10.6359) (-42.6919, 10.6359) knots 0 0 0 1 2 2 2
  spline S106 degree 2 poles (-42.6919, 10.6359) (-42.517, 10.6359) (-42.3008, 10.6935) (-42.235, 10.7409) knots 0 0 0 1 2 2 2
  spline S107 degree 2 poles (-42.235, 10.7409) (-42.1691, 10.7882) (-42.1074, 10.9323) (-42.1074, 11.0187) knots 0 0 0 1 2 2 2
  spline S108 degree 2 poles (-42.1074, 11.0187) (-42.1074, 11.0908) (-42.1691, 11.239) (-42.2309, 11.2843) knots 0 0 0 1 2 2 2
  spline S109 degree 2 poles (-42.2309, 11.2843) (-42.3029, 11.3357) (-42.5108, 11.3913) (-42.6919, 11.3913) knots 0 0 0 1 2 2 2
  line L83 (-41.7389, 12.9165) -> (-41.7389, 12.3196)
  line L84 (-41.7389, 12.3196) -> (-44.3921, 12.3196)
  line L85 (-44.3921, 12.3196) -> (-44.3921, 12.9165)
  line L86 (-44.3921, 12.9165) -> (-41.7389, 12.9165)
  point P0 (0, 0)
  point P1 (-42.7681, -14.3977)
  point P2 (-42.7681, -35.5)
  point P3 (-58.2681, 0)
  point P4 (-44.3921, 0)
  constraints: 4 midpoint, 1 horizontal alignment, 1 vertical alignment, 2 other
sketch "스케치15" plane through (14, 0, -35.5) normal (0, 0, -1) x (-1, 0, 0)
  line L0 (26.5, 33) -> (1.5, 33) projected
  line L1 (6.5, 30) -> (21.5, 30)
  line L2 (21.5, 30) -> (21.5, 33)
  line L3 (21.5, 33) -> (6.5, 33)
  line L4 (6.5, 33) -> (6.5, 30)
  line L5 (1.5, 31.5) -> (26.5, 31.5) projected
  line L6 (6.5, 30) -> (21.5, 33) construction
  line L7 (21.5, 30) -> (6.5, 33) construction
  point P0 (14, 0)
  point P1 (14, 31.5)
  dimension "d59" = 15
  constraints: 12 end point, 3 midpoint, 2 parallel, 1 horizontal, 1 perpendicular, 1 point on line
  measures "d59" distance of L3.end L2.end
extrude "돌출17" cut sketch "스케치15" against normal blind 10
extrude "돌출18" cut sketch "스케치8" along normal blind 12.5
sketch "스케치16" plane through (0, 33, 0) normal (0, 1, 0) x (1, 0, 0)
  line L0 (-11.25, -34.25) -> (11.25, -34.25)
  line L1 (14.25, -31.25) -> (14.25, 31.25)
  line L2 (11.25, 34.25) -> (-11.25, 34.25)
  line L3 (-14.25, 31.25) -> (-14.25, -31.25)
  line L4 (-14.25, -34.25) -> (14.25, 34.25) construction
  line L5 (14.25, -34.25) -> (-14.25, 34.25) construction
  arc A0 (-14.25, -31.25) -> (-11.25, -34.25) centre (-11.25, -31.25) ccw
  arc A1 (11.25, -34.25) -> (14.25, -31.25) centre (11.25, -31.25) ccw
  arc A2 (14.25, 31.25) -> (11.25, 34.25) centre (11.25, 31.25) ccw
  arc A3 (-11.25, 34.25) -> (-14.25, 31.25) centre (-11.25, 31.25) ccw
  point P0 (0, 0)
  dimension "d64" = 28.5
  dimension "d65" = 68.5
  dimension "d66" = 3
  constraints: 12 end point, 8 point on circle, 8 point on line, 8 tangent, 4 centre point, 3 equal radius, 2 midpoint, 2 parallel, 1 horizontal, 1 perpendicular
  measures "d64" distance of L5.end L4.end
  measures "d65" distance of L4.end L5.start
  measures "d66" radius of A0
extrude "돌출19" cut sketch "스케치16" against normal blind 1.5
extrude "돌출20" cut sketch "스케치14" against normal blind 10
extrude "돌출21" add sketch "스케치13" along normal blind 1.4
sketch "스케치18" plane through (0, 4.4, 0) normal (0, 1, 0) x (1, 0, 0)
  point P0 (0, 0)
